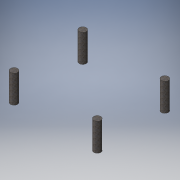
# Autodesk Inventor part: pylon
Saved by Autodesk Inventor 2016 (Build 200138000, 138)
## iProperties
Created: 2015-06-09
Part Number: pylon
Material: Concrete
Document SubType Name: Modeling
Designer: Haden
Density: 2.40731 g/cm^3
Appearance: Exposed Aggregate - Coarse
Author: Haden
Autodesk Inventor part; units mm, degrees
ref_plane "YZ Plane" through (0, 0, 0) normal (1, 0, 0) x (0, 1, 0)
ref_plane "XZ Plane" through (0, 0, 0) normal (0, 1, 0) x (-1, 0, 0)
ref_plane "XY Plane" through (0, 0, 0) normal (0, 0, 1) x (1, 0, 0)
sketch "Sketch1" plane through (0, 0, 0) normal (0, 1, 0) x (-1, 0, 0)
  circle A0 centre (0, 0) radius 152.4
  circle A1 centre (34.6834, -3000.1745) radius 152.4
  circle A2 centre (3695.0141, -3057.2118) radius 152.4
  circle A3 centre (3651.25, 0) radius 152.4
  dimension "d0" = 304.8
  dimension "d3" = 3651.25
  dimension "d4" = 3000.375
  dimension "d5" = 3057.525
  dimension "d6" = 3660.775
  dimension "d8" = 4699
  constraints: 4 centre point, 3 equal radius, 1 coincident, 1 horizontal alignment
  measures "d0" diameter of A0
  measures "d3" distance of point (0, 0) A3.centre
  measures "d4" distance of A1.centre point (0, 0)
  measures "d5" distance of A2.centre A3.centre
  measures "d6" distance of A1.centre A2.centre
  measures "d8" distance of A1.centre A3.centre
extrude "Extrusion2" add sketch "Sketch1" along normal blind 1219.2
body "Solid2"
